Autodesk Inventor part; units mm, degrees
(part 2 of 6)
  line L456 (38.3615, -15.9793) -> (38.1514, -15.9793) construction
  line L457 (38.1514, -15.9793) -> (38.3134, -15.1333) construction
  line L458 (38.3134, -15.1333) -> (38.3374, -15.0013) construction
  spline S134 degree 3 poles (38.3374, -15.0013) (38.3735, -14.7674) (38.3914, -14.4554) (38.5415, -14.2694) knots 58 58 58 58 59 59 59 59
  line L459 (38.3374, -15.0013) -> (38.3735, -14.7674) construction
  line L460 (38.3735, -14.7674) -> (38.3914, -14.4554) construction
  line L461 (38.3914, -14.4554) -> (38.5415, -14.2694) construction
  spline S135 degree 3 poles (38.5415, -14.2694) (38.5774, -14.2214) (38.985, -13.6999) (38.9854, -13.6994) knots 59 59 59 59 60 60 60 60
  line L462 (38.5415, -14.2694) -> (38.5774, -14.2214) construction
  line L463 (38.5774, -14.2214) -> (38.9854, -13.6994) construction
  line L464 (38.9854, -13.6994) -> (38.9854, -13.6994) construction
  spline S136 degree 3 poles (38.9854, -13.6994) (38.9734, -13.6934) (38.9255, -13.7534) (38.8954, -13.7894) knots 60 60 60 60 61 61 61 61
  line L465 (38.9854, -13.6994) -> (38.9734, -13.6934) construction
  line L466 (38.9734, -13.6934) -> (38.9255, -13.7534) construction
  line L467 (38.9255, -13.7534) -> (38.8954, -13.7894) construction
  spline S137 degree 3 poles (38.8954, -13.7894) (38.8954, -13.7954) (38.8895, -13.8014) (38.8894, -13.8014) knots 61 61 61 61 62 62 62 62
  line L468 (38.8954, -13.7894) -> (38.8954, -13.7954) construction
  line L469 (38.8954, -13.7954) -> (38.8894, -13.8014) construction
  line L470 (38.8894, -13.8014) -> (38.8894, -13.8014) construction
  spline S138 degree 3 poles (38.8894, -13.8014) (38.8835, -13.8134) (38.8774, -13.8194) (38.8774, -13.8194) knots 62 62 62 62 63 63 63 63
  line L471 (38.8894, -13.8014) -> (38.8835, -13.8134) construction
  line L472 (38.8835, -13.8134) -> (38.8774, -13.8194) construction
  line L473 (38.8774, -13.8194) -> (38.8774, -13.8194) construction
  spline S139 degree 3 poles (38.8774, -13.8194) (38.8774, -13.8134) (38.8835, -13.8074) (38.8894, -13.8014) knots 63 63 63 63 64 64 64 64
  line L474 (38.8774, -13.8194) -> (38.8774, -13.8134) construction
  line L475 (38.8774, -13.8134) -> (38.8835, -13.8074) construction
  line L476 (38.8835, -13.8074) -> (38.8894, -13.8014) construction
  line L477 (38.8894, -13.8014) -> (38.8954, -13.7894)
  line L478 (38.8954, -13.7894) -> (39.1534, -13.4414)
  line L479 (39.1534, -13.4414) -> (39.1714, -13.4174)
  line L480 (39.1714, -13.4174) -> (39.2194, -13.3514)
  spline S140 degree 3 poles (39.2194, -13.3514) (39.2254, -13.3574) (39.2194, -13.3694) (39.2134, -13.3814) knots 68 68 68 68 69 69 69 69
  line L481 (39.2194, -13.3514) -> (39.2254, -13.3574) construction
  line L482 (39.2254, -13.3574) -> (39.2194, -13.3694) construction
  line L483 (39.2194, -13.3694) -> (39.2134, -13.3814) construction
  line L484 (39.2134, -13.3814) -> (39.2675, -13.3214)
  line L485 (39.2675, -13.3214) -> (39.4234, -13.1174)
  spline S141 degree 3 poles (39.4234, -13.1174) (39.5374, -12.9554) (39.6454, -12.7814) (39.7474, -12.6134) knots 71 71 71 71 72 72 72 72
  line L486 (39.4234, -13.1174) -> (39.5374, -12.9554) construction
  line L487 (39.5374, -12.9554) -> (39.6454, -12.7814) construction
  line L488 (39.6454, -12.7814) -> (39.7474, -12.6134) construction
  spline S142 degree 3 poles (39.7474, -12.6134) (39.9094, -12.3374) (40.1314, -11.9414) (40.0114, -11.6054) knots 72 72 72 72 73 73 73 73
  line L489 (39.7474, -12.6134) -> (39.9094, -12.3374) construction
  line L490 (39.9094, -12.3374) -> (40.1314, -11.9414) construction
  line L491 (40.1314, -11.9414) -> (40.0114, -11.6054) construction
  spline S143 degree 3 poles (40.0114, -11.6054) (39.9214, -11.3594) (39.5914, -11.3114) (39.3694, -11.3954) knots 73 73 73 73 74 74 74 74
  line L492 (40.0114, -11.6054) -> (39.9214, -11.3594) construction
  line L493 (39.9214, -11.3594) -> (39.5914, -11.3114) construction
  line L494 (39.5914, -11.3114) -> (39.3694, -11.3954) construction
  spline S144 degree 3 poles (39.3694, -11.3954) (39.2074, -11.4554) (39.0695, -11.5814) (38.9554, -11.7134) knots 74 74 74 74 75 75 75 75
  line L495 (39.3694, -11.3954) -> (39.2074, -11.4554) construction
  line L496 (39.2074, -11.4554) -> (39.0695, -11.5814) construction
  line L497 (39.0695, -11.5814) -> (38.9554, -11.7134) construction
  spline S145 degree 3 poles (38.9554, -11.7134) (38.8954, -11.7914) (38.8354, -11.8769) (38.7815, -11.9669) knots 75 75 75 75 76 76 76 76
  line L498 (38.9554, -11.7134) -> (38.8954, -11.7914) construction
  line L499 (38.8954, -11.7914) -> (38.8354, -11.8769) construction
  line L500 (38.8354, -11.8769) -> (38.7815, -11.9669) construction
  spline S146 degree 3 poles (38.7815, -11.9669) (38.7634, -11.9909) (38.6855, -12.1667) (38.6674, -12.2083) knots 76 76 76 76 77 77 77 77
  line L501 (38.7815, -11.9669) -> (38.7634, -11.9909) construction
  line L502 (38.7634, -11.9909) -> (38.6855, -12.1667) construction
  line L503 (38.6855, -12.1667) -> (38.6674, -12.2083) construction
  line L504 (38.6674, -12.2083) -> (38.6735, -12.2083)
  spline S147 degree 3 poles (38.6735, -12.2083) (38.6375, -12.2917) (38.6014, -12.3389) (38.5774, -12.4049) knots 78 78 78 78 79 79 79 79
  line L505 (38.6735, -12.2083) -> (38.6375, -12.2917) construction
  line L506 (38.6375, -12.2917) -> (38.6014, -12.3389) construction
  line L507 (38.6014, -12.3389) -> (38.5774, -12.4049) construction
  spline S148 degree 3 poles (38.5774, -12.4049) (38.5894, -12.3569) (38.6195, -12.2601) (38.6434, -12.2421) knots 79 79 79 79 80 80 80 80
  line L508 (38.5774, -12.4049) -> (38.5894, -12.3569) construction
  line L509 (38.5894, -12.3569) -> (38.6195, -12.2601) construction
  line L510 (38.6195, -12.2601) -> (38.6434, -12.2421) construction
  spline S149 degree 3 poles (38.6434, -12.2421) (38.5955, -12.2781) (38.5535, -12.4518) (38.5415, -12.4698) knots 80 80 80 80 81 81 81 81
  line L511 (38.6434, -12.2421) -> (38.5955, -12.2781) construction
  line L512 (38.5955, -12.2781) -> (38.5535, -12.4518) construction
  line L513 (38.5535, -12.4518) -> (38.5415, -12.4698) construction
  spline S150 degree 3 poles (38.5415, -12.4698) (38.3134, -12.9678) (38.1155, -13.4716) (37.9715, -13.9996) knots 81 81 81 81 82 82 82 82
  line L514 (38.5415, -12.4698) -> (38.3134, -12.9678) construction
  line L515 (38.3134, -12.9678) -> (38.1155, -13.4716) construction
  line L516 (38.1155, -13.4716) -> (37.9715, -13.9996) construction
  spline S151 degree 3 poles (37.9715, -13.9996) (37.8094, -13.8136) (37.5515, -13.4955) (37.2695, -13.6095) knots 82 82 82 82 83 83 83 83
  line L517 (37.9715, -13.9996) -> (37.8094, -13.8136) construction
  line L518 (37.8094, -13.8136) -> (37.5515, -13.4955) construction
  line L519 (37.5515, -13.4955) -> (37.2695, -13.6095) construction
  spline S152 degree 3 poles (37.2695, -13.6095) (37.0355, -13.7054) (36.8615, -13.9514) (36.7415, -14.1674) knots 83 83 83 83 84 84 84 84
  line L520 (37.2695, -13.6095) -> (37.0355, -13.7054) construction
  line L521 (37.0355, -13.7054) -> (36.8615, -13.9514) construction
  line L522 (36.8615, -13.9514) -> (36.7415, -14.1674) construction
  spline S153 degree 3 poles (36.7415, -14.1674) (36.7197, -14.2061) (36.7017, -14.2451) (36.6852, -14.2842) knots 84 84 84 84 85 85 85 85
  line L523 (36.7415, -14.1674) -> (36.7197, -14.2061) construction
  line L524 (36.7197, -14.2061) -> (36.7017, -14.2451) construction
  line L525 (36.7017, -14.2451) -> (36.6852, -14.2842) construction
  spline S154 degree 3 poles (36.6852, -14.2842) (36.6202, -14.3421) (36.5497, -14.3987) (36.4895, -14.4554) knots 85 85 85 85 86 86 86 86
  line L526 (36.6852, -14.2842) -> (36.6202, -14.3421) construction
  line L527 (36.6202, -14.3421) -> (36.5497, -14.3987) construction
  line L528 (36.5497, -14.3987) -> (36.4895, -14.4554) construction
  spline S155 degree 3 poles (36.4895, -14.4554) (36.3515, -14.5754) (36.2135, -14.7014) (36.0695, -14.8153) knots 86 86 86 86 87 87 87 87
  line L529 (36.4895, -14.4554) -> (36.3515, -14.5754) construction
  line L530 (36.3515, -14.5754) -> (36.2135, -14.7014) construction
  line L531 (36.2135, -14.7014) -> (36.0695, -14.8153) construction
  spline S156 degree 3 poles (36.0695, -14.8153) (35.9975, -14.8753) (35.9075, -14.9594) (35.8175, -14.9893) knots 87 87 87 87 88 88 88 88
  line L532 (36.0695, -14.8153) -> (35.9975, -14.8753) construction
  line L533 (35.9975, -14.8753) -> (35.9075, -14.9594) construction
  line L534 (35.9075, -14.9594) -> (35.8175, -14.9893) construction
  spline S157 degree 3 poles (35.8175, -14.9893) (35.8055, -14.9953) (35.7635, -15.0013) (35.7635, -15.0073) knots 88 88 88 88 89 89 89 89
  line L535 (35.8175, -14.9893) -> (35.8055, -14.9953) construction
  line L536 (35.8055, -14.9953) -> (35.7635, -15.0013) construction
  line L537 (35.7635, -15.0013) -> (35.7635, -15.0073) construction
  line L538 (35.7635, -15.0073) -> (35.7575, -15.0013)
  spline S158 degree 3 poles (35.7575, -15.0013) (35.7575, -15.0012) (35.7515, -14.9054) (35.7575, -14.8994) knots 90 90 90 90 91 91 91 91
  line L539 (35.7575, -15.0013) -> (35.7575, -15.0013) construction
  line L540 (35.7575, -15.0013) -> (35.7515, -14.9054) construction
  line L541 (35.7515, -14.9054) -> (35.7575, -14.8994) construction
  spline S159 degree 3 poles (35.7575, -14.8994) (35.7635, -14.8214) (35.7875, -14.7433) (35.8115, -14.6713) knots 91 91 91 91 92 92 92 92
  line L542 (35.7575, -14.8994) -> (35.7635, -14.8214) construction
  line L543 (35.7635, -14.8214) -> (35.7875, -14.7433) construction
  line L544 (35.7875, -14.7433) -> (35.8115, -14.6713) construction
  spline S160 degree 3 poles (35.8115, -14.6713) (35.8175, -14.6593) (35.8835, -14.4554) (35.8715, -14.4554) knots 92 92 92 92 93 93 93 93
  line L545 (35.8115, -14.6713) -> (35.8175, -14.6593) construction
  line L546 (35.8175, -14.6593) -> (35.8835, -14.4554) construction
  line L547 (35.8835, -14.4554) -> (35.8715, -14.4554) construction
  line L548 (35.8715, -14.4554) -> (35.8415, -14.4914)
  spline S161 degree 3 poles (35.8415, -14.4914) (35.8775, -14.4194) (35.9255, -14.3474) (35.9675, -14.2694) knots 94 94 94 94 95 95 95 95
  line L549 (35.8415, -14.4914) -> (35.8775, -14.4194) construction
  line L550 (35.8775, -14.4194) -> (35.9255, -14.3474) construction
  line L551 (35.9255, -14.3474) -> (35.9675, -14.2694) construction
  spline S162 degree 3 poles (35.9675, -14.2694) (35.8715, -14.3594) (35.8055, -14.4614) (35.7575, -14.5874) knots 95 95 95 95 96 96 96 96
  line L552 (35.9675, -14.2694) -> (35.8715, -14.3594) construction
  line L553 (35.8715, -14.3594) -> (35.8055, -14.4614) construction
  line L554 (35.8055, -14.4614) -> (35.7575, -14.5874) construction
  spline S163 degree 3 poles (35.7575, -14.5874) (35.7335, -14.6474) (35.6675, -14.7554) (35.6555, -14.8454) knots 96 96 96 96 97 97 97 97
  line L555 (35.7575, -14.5874) -> (35.7335, -14.6474) construction
  line L556 (35.7335, -14.6474) -> (35.6675, -14.7554) construction
  line L557 (35.6675, -14.7554) -> (35.6555, -14.8454) construction
  spline S164 degree 3 poles (35.6555, -14.8454) (35.6675, -14.7134) (35.7575, -14.5393) (35.7995, -14.4614) knots 97 97 97 97 98 98 98 98
  line L558 (35.6555, -14.8454) -> (35.6675, -14.7134) construction
  line L559 (35.6675, -14.7134) -> (35.7575, -14.5393) construction
  line L560 (35.7575, -14.5393) -> (35.7995, -14.4614) construction
  spline S165 degree 3 poles (35.7995, -14.4614) (35.8595, -14.3354) (35.9255, -14.1914) (36.0035, -14.0714) knots 98 98 98 98 99 99 99 99
  line L561 (35.7995, -14.4614) -> (35.8595, -14.3354) construction
  line L562 (35.8595, -14.3354) -> (35.9255, -14.1914) construction
  line L563 (35.9255, -14.1914) -> (36.0035, -14.0714) construction
  spline S166 degree 3 poles (36.0035, -14.0714) (36.1475, -13.8554) (36.4595, -13.6574) (36.3635, -13.3574) knots 99 99 99 99 100 100 100 100
  line L564 (36.0035, -14.0714) -> (36.1475, -13.8554) construction
  line L565 (36.1475, -13.8554) -> (36.4595, -13.6574) construction
  line L566 (36.4595, -13.6574) -> (36.3635, -13.3574) construction
  spline S167 degree 3 poles (36.3635, -13.3574) (36.2795, -13.0754) (36.0575, -13.0694) (35.8835, -13.2314) knots 100 100 100 100 101 101 101 101
  line L567 (36.3635, -13.3574) -> (36.2795, -13.0754) construction
  line L568 (36.2795, -13.0754) -> (36.0575, -13.0694) construction
  line L569 (36.0575, -13.0694) -> (35.8835, -13.2314) construction
  spline S168 degree 3 poles (35.8835, -13.2314) (35.7995, -13.3094) (35.0855, -14.2214) (35.1036, -14.2334) knots 101 101 101 101 102 102 102 102
  line L570 (35.8835, -13.2314) -> (35.7995, -13.3094) construction
  line L571 (35.7995, -13.3094) -> (35.0855, -14.2214) construction
  line L572 (35.0855, -14.2214) -> (35.1036, -14.2334) construction
  spline S169 degree 3 poles (35.1036, -14.2334) (35.1036, -14.2333) (35.1635, -14.1614) (35.2415, -14.0594) knots 102 102 102 102 103 103 103 103
  line L573 (35.1036, -14.2334) -> (35.1036, -14.2334) construction
  line L574 (35.1036, -14.2334) -> (35.1635, -14.1614) construction
  line L575 (35.1635, -14.1614) -> (35.2415, -14.0594) construction
  line L576 (35.2415, -14.0594) -> (34.8875, -14.5754)
  spline S170 degree 3 poles (34.8875, -14.5754) (34.8816, -14.5754) (34.9476, -14.4733) (34.9415, -14.4673) knots 104 104 104 104 105 105 105 105
  line L577 (34.8875, -14.5754) -> (34.8816, -14.5754) construction
  line L578 (34.8816, -14.5754) -> (34.9476, -14.4733) construction
  line L579 (34.9476, -14.4733) -> (34.9415, -14.4673) construction
  spline S171 degree 3 poles (34.9415, -14.4673) (34.9355, -14.4614) (34.8936, -14.5034) (34.8875, -14.5273) knots 105 105 105 105 106 106 106 106
  line L580 (34.9415, -14.4673) -> (34.9355, -14.4614) construction
  line L581 (34.9355, -14.4614) -> (34.8936, -14.5034) construction
  line L582 (34.8936, -14.5034) -> (34.8875, -14.5273) construction
  spline S172 degree 3 poles (34.8875, -14.5273) (34.8995, -14.4013) (34.9415, -14.2753) (34.9535, -14.1494) knots 106 106 106 106 107 107 107 107
  line L583 (34.8875, -14.5273) -> (34.8995, -14.4013) construction
  line L584 (34.8995, -14.4013) -> (34.9415, -14.2753) construction
  line L585 (34.9415, -14.2753) -> (34.9535, -14.1494) construction
  spline S173 degree 3 poles (34.9535, -14.1494) (34.9596, -14.1014) (34.9535, -14.0654) (34.9655, -14.0174) knots 107 107 107 107 108 108 108 108
  line L586 (34.9535, -14.1494) -> (34.9596, -14.1014) construction
  line L587 (34.9596, -14.1014) -> (34.9535, -14.0654) construction
  line L588 (34.9535, -14.0654) -> (34.9655, -14.0174) construction
  spline S174 degree 3 poles (34.9655, -14.0174) (34.9895, -13.9394) (35.0135, -13.8554) (35.0496, -13.7894) knots 108 108 108 108 109 109 109 109
  line L589 (34.9655, -14.0174) -> (34.9895, -13.9394) construction
  line L590 (34.9895, -13.9394) -> (35.0135, -13.8554) construction
  line L591 (35.0135, -13.8554) -> (35.0496, -13.7894) construction
  spline S175 degree 3 poles (35.0496, -13.7894) (35.0735, -13.7414) (35.1215, -13.6994) (35.1335, -13.6514) knots 109 109 109 109 110 110 110 110
  line L592 (35.0496, -13.7894) -> (35.0735, -13.7414) construction
  line L593 (35.0735, -13.7414) -> (35.1215, -13.6994) construction
  line L594 (35.1215, -13.6994) -> (35.1335, -13.6514) construction
  spline S176 degree 3 poles (35.1335, -13.6514) (35.1576, -13.5734) (35.1515, -13.5434) (35.2055, -13.4774) knots 110 110 110 110 111 111 111 111
  line L595 (35.1335, -13.6514) -> (35.1576, -13.5734) construction
  line L596 (35.1576, -13.5734) -> (35.1515, -13.5434) construction
  line L597 (35.1515, -13.5434) -> (35.2055, -13.4774) construction
  spline S177 degree 3 poles (35.2055, -13.4774) (35.2535, -13.4174) (35.3255, -13.3574) (35.3676, -13.3034) knots 111 111 111 111 112 112 112 112
  line L598 (35.2055, -13.4774) -> (35.2535, -13.4174) construction
  line L599 (35.2535, -13.4174) -> (35.3255, -13.3574) construction
  line L600 (35.3255, -13.3574) -> (35.3676, -13.3034) construction
  spline S178 degree 3 poles (35.3676, -13.3034) (35.4695, -13.1534) (35.2955, -13.0514) (35.1995, -13.0334) knots 112 112 112 112 113 113 113 113
  line L601 (35.3676, -13.3034) -> (35.4695, -13.1534) construction
  line L602 (35.4695, -13.1534) -> (35.2955, -13.0514) construction
  line L603 (35.2955, -13.0514) -> (35.1995, -13.0334) construction
  spline S179 degree 3 poles (35.1995, -13.0334) (35.1215, -13.0214) (35.0435, -13.0154) (34.9716, -13.0574) knots 113 113 113 113 114 114 114 114
  line L604 (35.1995, -13.0334) -> (35.1215, -13.0214) construction
  line L605 (35.1215, -13.0214) -> (35.0435, -13.0154) construction
  line L606 (35.0435, -13.0154) -> (34.9716, -13.0574) construction
  spline S180 degree 3 poles (34.9716, -13.0574) (34.8936, -13.1054) (34.9115, -13.1474) (34.8936, -13.2134) knots 114 114 114 114 115 115 115 115
  line L607 (34.9716, -13.0574) -> (34.8936, -13.1054) construction
  line L608 (34.8936, -13.1054) -> (34.9115, -13.1474) construction
  line L609 (34.9115, -13.1474) -> (34.8936, -13.2134) construction
  spline S181 degree 3 poles (34.8936, -13.2134) (34.8755, -13.2974) (34.8156, -13.3934) (34.7856, -13.4714) knots 115 115 115 115 116 116 116 116
  line L610 (34.8936, -13.2134) -> (34.8755, -13.2974) construction
  line L611 (34.8755, -13.2974) -> (34.8156, -13.3934) construction
  line L612 (34.8156, -13.3934) -> (34.7856, -13.4714) construction
  spline S182 degree 3 poles (34.7856, -13.4714) (34.7375, -13.5974) (34.6956, -13.7234) (34.6536, -13.8494) knots 116 116 116 116 117 117 117 117
  line L613 (34.7856, -13.4714) -> (34.7375, -13.5974) construction
  line L614 (34.7375, -13.5974) -> (34.6956, -13.7234) construction
  line L615 (34.6956, -13.7234) -> (34.6536, -13.8494) construction
  spline S183 degree 3 poles (34.6536, -13.8494) (34.6056, -13.9754) (34.5575, -14.0954) (34.5216, -14.2214) knots 117 117 117 117 118 118 118 118
  line L616 (34.6536, -13.8494) -> (34.6056, -13.9754) construction
  line L617 (34.6056, -13.9754) -> (34.5575, -14.0954) construction
  line L618 (34.5575, -14.0954) -> (34.5216, -14.2214) construction
  spline S184 degree 3 poles (34.5216, -14.2214) (34.4915, -14.3234) (34.4976, -14.4194) (34.4856, -14.5154) knots 118 118 118 118 119 119 119 119
  line L619 (34.5216, -14.2214) -> (34.4915, -14.3234) construction
  line L620 (34.4915, -14.3234) -> (34.4976, -14.4194) construction
  line L621 (34.4976, -14.4194) -> (34.4856, -14.5154) construction
  spline S185 degree 3 poles (34.4856, -14.5154) (34.4815, -14.5514) (34.4771, -14.5833) (34.4746, -14.6136) knots 119 119 119 119 120 120 120 120
  line L622 (34.4856, -14.5154) -> (34.4815, -14.5514) construction
  line L623 (34.4815, -14.5514) -> (34.4771, -14.5833) construction
  line L624 (34.4771, -14.5833) -> (34.4746, -14.6136) construction
  spline S186 degree 3 poles (34.4746, -14.6136) (34.3338, -14.8266) (34.1908, -15.0385) (34.0296, -15.2413) knots 120 120 120 120 121 121 121 121
  line L625 (34.4746, -14.6136) -> (34.3338, -14.8266) construction
  line L626 (34.3338, -14.8266) -> (34.1908, -15.0385) construction
  line L627 (34.1908, -15.0385) -> (34.0296, -15.2413) construction
  spline S187 degree 3 poles (34.0296, -15.2413) (33.4116, -16.0033) (33.8436, -14.6474) (33.7956, -14.6593) knots 121 121 121 121 122 122 122 122
  line L628 (34.0296, -15.2413) -> (33.4116, -16.0033) construction
  line L629 (33.4116, -16.0033) -> (33.8436, -14.6474) construction
  line L630 (33.8436, -14.6474) -> (33.7956, -14.6593) construction
  spline S188 degree 3 poles (33.7956, -14.6593) (33.7716, -14.6653) (33.7536, -14.7554) (33.7476, -14.7734) knots 122 122 122 122 123 123 123 123
  line L631 (33.7956, -14.6593) -> (33.7716, -14.6653) construction
  line L632 (33.7716, -14.6653) -> (33.7536, -14.7554) construction
  line L633 (33.7536, -14.7554) -> (33.7476, -14.7734) construction
  spline S189 degree 3 poles (33.7476, -14.7734) (33.7956, -14.5574) (33.8856, -14.2994) (33.9996, -14.0894) knots 123 123 123 123 124 124 124 124
  line L634 (33.7476, -14.7734) -> (33.7956, -14.5574) construction
  line L635 (33.7956, -14.5574) -> (33.8856, -14.2994) construction
  line L636 (33.8856, -14.2994) -> (33.9996, -14.0894) construction
  spline S190 degree 3 poles (33.9996, -14.0894) (34.0656, -13.9574) (34.1436, -13.8494) (34.0236, -13.7054) knots 124 124 124 124 125 125 125 125
  line L637 (33.9996, -14.0894) -> (34.0656, -13.9574) construction
  line L638 (34.0656, -13.9574) -> (34.1436, -13.8494) construction
  line L639 (34.1436, -13.8494) -> (34.0236, -13.7054) construction
  spline S191 degree 3 poles (34.0236, -13.7054) (33.8016, -13.4354) (33.5436, -13.6814) (33.3996, -13.8674) knots 125 125 125 125 126 126 126 126
  line L640 (34.0236, -13.7054) -> (33.8016, -13.4354) construction
  line L641 (33.8016, -13.4354) -> (33.5436, -13.6814) construction
  line L642 (33.5436, -13.6814) -> (33.3996, -13.8674) construction
  spline S192 degree 3 poles (33.3996, -13.8674) (33.3396, -13.6394) (33.2196, -13.3034) (32.9256, -13.3034) (32.7936, -13.3034) (32.7156, -13.3694) (32.6256, -13.4474) knots 126 126 126 126 127 127 127 128 128 128 128
  line L643 (33.3996, -13.8674) -> (33.3396, -13.6394) construction
  line L644 (33.3396, -13.6394) -> (33.2196, -13.3034) construction
  line L645 (33.2196, -13.3034) -> (32.9256, -13.3034) construction
  line L646 (32.9256, -13.3034) -> (32.7936, -13.3034) construction
  line L647 (32.7936, -13.3034) -> (32.7156, -13.3694) construction
  line L648 (32.7156, -13.3694) -> (32.6256, -13.4474) construction
  spline S193 degree 3 poles (32.6256, -13.4474) (32.5716, -13.4834) (32.5296, -13.4894) (32.4816, -13.5314) knots 128 128 128 128 129 129 129 129
  line L649 (32.6256, -13.4474) -> (32.5716, -13.4834) construction
  line L650 (32.5716, -13.4834) -> (32.5296, -13.4894) construction
  line L651 (32.5296, -13.4894) -> (32.4816, -13.5314) construction
  spline S194 degree 3 poles (32.4816, -13.5314) (32.4036, -13.5854) (32.3496, -13.6694) (32.2956, -13.7414) knots 129 129 129 129 130 130 130 130
  line L652 (32.4816, -13.5314) -> (32.4036, -13.5854) construction
  line L653 (32.4036, -13.5854) -> (32.3496, -13.6694) construction
  line L654 (32.3496, -13.6694) -> (32.2956, -13.7414) construction
  spline S195 degree 3 poles (32.2956, -13.7414) (32.0916, -14.0414) (31.9476, -14.4194) (31.8816, -14.7674) knots 130 130 130 130 131 131 131 131
  line L655 (32.2956, -13.7414) -> (32.0916, -14.0414) construction
  line L656 (32.0916, -14.0414) -> (31.9476, -14.4194) construction
  line L657 (31.9476, -14.4194) -> (31.8816, -14.7674) construction
  spline S196 degree 3 poles (31.8816, -14.7674) (31.8516, -14.9353) (31.8396, -15.1213) (31.8876, -15.2893) knots 131 131 131 131 132 132 132 132
  line L658 (31.8816, -14.7674) -> (31.8516, -14.9353) construction
  line L659 (31.8516, -14.9353) -> (31.8396, -15.1213) construction
  line L660 (31.8396, -15.1213) -> (31.8876, -15.2893) construction
  spline S197 degree 3 poles (31.8876, -15.2893) (31.9176, -15.3853) (32.0256, -15.6013) (32.1636, -15.5833) knots 132 132 132 132 133 133 133 133
  line L661 (31.8876, -15.2893) -> (31.9176, -15.3853) construction
  line L662 (31.9176, -15.3853) -> (32.0256, -15.6013) construction
  line L663 (32.0256, -15.6013) -> (32.1636, -15.5833) construction
  spline S198 degree 3 poles (32.1636, -15.5833) (32.1696, -15.5833) (32.1576, -15.5773) (32.1396, -15.5653) knots 133 133 133 133 134 134 134 134
  line L664 (32.1636, -15.5833) -> (32.1696, -15.5833) construction
  line L665 (32.1696, -15.5833) -> (32.1576, -15.5773) construction
  line L666 (32.1576, -15.5773) -> (32.1396, -15.5653) construction
  spline S199 degree 3 poles (32.1396, -15.5653) (32.2236, -15.5893) (32.3196, -15.5773) (32.3916, -15.5293) knots 134 134 134 134 135 135 135 135
  line L667 (32.1396, -15.5653) -> (32.2236, -15.5893) construction
  line L668 (32.2236, -15.5893) -> (32.3196, -15.5773) construction
  line L669 (32.3196, -15.5773) -> (32.3916, -15.5293) construction
  spline S200 degree 3 poles (32.3916, -15.5293) (32.3976, -15.5413) (32.3257, -15.5713) (32.3256, -15.5713) knots 135 135 135 135 136 136 136 136
  line L670 (32.3916, -15.5293) -> (32.3976, -15.5413) construction
  line L671 (32.3976, -15.5413) -> (32.3256, -15.5713) construction
  line L672 (32.3256, -15.5713) -> (32.3256, -15.5713) construction
  spline S201 degree 3 poles (32.3256, -15.5713) (32.3916, -15.6733) (32.8836, -15.0793) (32.9196, -15.0253) knots 136 136 136 136 137 137 137 137
  line L673 (32.3256, -15.5713) -> (32.3916, -15.6733) construction
  line L674 (32.3916, -15.6733) -> (32.8836, -15.0793) construction
  line L675 (32.8836, -15.0793) -> (32.9196, -15.0253) construction
  spline S202 degree 3 poles (32.9196, -15.0253) (32.9976, -14.9173) (33.0516, -14.8033) (33.1236, -14.6894) knots 137 137 137 137 138 138 138 138
  line L676 (32.9196, -15.0253) -> (32.9976, -14.9173) construction
  line L677 (32.9976, -14.9173) -> (33.0516, -14.8033) construction
  line L678 (33.0516, -14.8033) -> (33.1236, -14.6894) construction
  spline S203 degree 3 poles (33.1236, -14.6894) (33.1776, -14.6053) (33.2616, -14.4974) (33.3216, -14.4073) knots 138 138 138 138 139 139 139 139
  line L679 (33.1236, -14.6894) -> (33.1776, -14.6053) construction
  line L680 (33.1776, -14.6053) -> (33.2616, -14.4974) construction
  line L681 (33.2616, -14.4974) -> (33.3216, -14.4073) construction
  spline S204 degree 3 poles (33.3216, -14.4073) (33.3156, -14.4494) (33.3156, -14.5033) (33.3156, -14.5034) knots 139 139 139 139 140 140 140 140
  line L682 (33.3216, -14.4073) -> (33.3156, -14.4494) construction
  line L683 (33.3156, -14.4494) -> (33.3156, -14.5034) construction
  line L684 (33.3156, -14.5034) -> (33.3156, -14.5034) construction
  spline S205 degree 3 poles (33.3156, -14.5034) (33.2076, -14.8454) (33.1056, -15.2173) (33.2496, -15.5713) knots 140 140 140 140 141 141 141 141
  line L685 (33.3156, -14.5034) -> (33.2076, -14.8454) construction
  line L686 (33.2076, -14.8454) -> (33.1056, -15.2173) construction
  line L687 (33.1056, -15.2173) -> (33.2496, -15.5713) construction
  spline S206 degree 3 poles (33.2496, -15.5713) (33.3156, -15.7513) (33.4776, -15.9193) (33.6816, -15.8833) knots 141 141 141 141 142 142 142 142
  line L688 (33.2496, -15.5713) -> (33.3156, -15.7513) construction
  line L689 (33.3156, -15.7513) -> (33.4776, -15.9193) construction
  line L690 (33.4776, -15.9193) -> (33.6816, -15.8833) construction
  spline S207 degree 3 poles (33.6816, -15.8833) (33.8616, -15.8533) (34.0116, -15.6793) (34.1196, -15.5413) knots 142 142 142 142 143 143 143 143
  line L691 (33.6816, -15.8833) -> (33.8616, -15.8533) construction
  line L692 (33.8616, -15.8533) -> (34.0116, -15.6793) construction
  line L693 (34.0116, -15.6793) -> (34.1196, -15.5413) construction
  spline S208 degree 3 poles (34.1196, -15.5413) (34.2516, -15.3853) (34.3656, -15.2113) (34.4796, -15.0314) knots 143 143 143 143 144 144 144 144
  line L694 (34.1196, -15.5413) -> (34.2516, -15.3853) construction
  line L695 (34.2516, -15.3853) -> (34.3656, -15.2113) construction
  line L696 (34.3656, -15.2113) -> (34.4796, -15.0314) construction
  spline S209 degree 3 poles (34.4796, -15.0314) (34.5108, -14.9786) (34.5411, -14.9256) (34.5709, -14.8722) knots 144 144 144 144 145 145 145 145
  line L697 (34.4796, -15.0314) -> (34.5108, -14.9786) construction
  line L698 (34.5108, -14.9786) -> (34.5411, -14.9256) construction
  line L699 (34.5411, -14.9256) -> (34.5709, -14.8722) construction
  spline S210 degree 3 poles (34.5709, -14.8722) (34.6468, -14.9531) (34.7584, -15.0165) (34.8396, -14.9173) knots 145 145 145 145 146 146 146 146
  line L700 (34.5709, -14.8722) -> (34.6468, -14.9531) construction
  line L701 (34.6468, -14.9531) -> (34.7584, -15.0165) construction
  line L702 (34.7584, -15.0165) -> (34.8396, -14.9173) construction
  line L703 (34.8396, -14.9173) -> (34.8635, -14.9654)
  spline S211 degree 3 poles (34.8635, -14.9654) (34.9655, -14.7433) (35.1215, -14.5453) (35.2475, -14.3294) knots 147 147 147 147 148 148 148 148
  line L704 (34.8635, -14.9654) -> (34.9655, -14.7433) construction
  line L705 (34.9655, -14.7433) -> (35.1215, -14.5453) construction
  line L706 (35.1215, -14.5453) -> (35.2475, -14.3294) construction
  spline S212 degree 3 poles (35.2475, -14.3294) (35.3016, -14.2334) (35.3975, -14.1674) (35.4755, -14.0654) knots 148 148 148 148 149 149 149 149
  line L707 (35.2475, -14.3294) -> (35.3016, -14.2334) construction
  line L708 (35.3016, -14.2334) -> (35.3975, -14.1674) construction
  line L709 (35.3975, -14.1674) -> (35.4755, -14.0654) construction
  spline S213 degree 3 poles (35.4755, -14.0654) (35.5835, -13.9214) (35.6795, -13.7774) (35.7995, -13.6394) knots 149 149 149 149 150 150 150 150
  line L710 (35.4755, -14.0654) -> (35.5835, -13.9214) construction
  line L711 (35.5835, -13.9214) -> (35.6795, -13.7774) construction
  line L712 (35.6795, -13.7774) -> (35.7995, -13.6394) construction
  spline S214 degree 3 poles (35.7995, -13.6394) (35.7815, -13.6694) (35.7035, -13.8074) (35.7095, -13.8134) knots 150 150 150 150 151 151 151 151
  line L713 (35.7995, -13.6394) -> (35.7815, -13.6694) construction
  line L714 (35.7815, -13.6694) -> (35.7035, -13.8074) construction
  line L715 (35.7035, -13.8074) -> (35.7095, -13.8134) construction
  spline S215 degree 3 poles (35.7095, -13.8134) (35.7215, -13.8074) (35.7275, -13.7954) (35.7395, -13.7834) knots 151 151 151 151 152 152 152 152
  line L716 (35.7095, -13.8134) -> (35.7215, -13.8074) construction
  line L717 (35.7215, -13.8074) -> (35.7275, -13.7954) construction
  line L718 (35.7275, -13.7954) -> (35.7395, -13.7834) construction
  line L719 (35.7395, -13.7834) -> (35.6555, -13.9514)
  spline S216 degree 3 poles (35.6555, -13.9514) (35.6495, -13.9454) (35.6795, -13.9034) (35.6675, -13.9034) knots 153 153 153 153 154 154 154 154
  line L720 (35.6555, -13.9514) -> (35.6495, -13.9454) construction
  line L721 (35.6495, -13.9454) -> (35.6795, -13.9034) construction
  line L722 (35.6795, -13.9034) -> (35.6675, -13.9034) construction
  spline S217 degree 3 poles (35.6675, -13.9034) (35.6255, -13.8914) (35.4995, -14.2274) (35.4875, -14.2574) knots 154 154 154 154 155 155 155 155
  line L723 (35.6675, -13.9034) -> (35.6255, -13.8914) construction
  line L724 (35.6255, -13.8914) -> (35.4995, -14.2274) construction
  line L725 (35.4995, -14.2274) -> (35.4875, -14.2574) construction
  spline S218 degree 3 poles (35.4875, -14.2574) (35.4455, -14.3894) (35.4395, -14.5094) (35.4275, -14.6474) knots 155 155 155 155 156 156 156 156
  line L726 (35.4875, -14.2574) -> (35.4455, -14.3894) construction
  line L727 (35.4455, -14.3894) -> (35.4395, -14.5094) construction
  line L728 (35.4395, -14.5094) -> (35.4275, -14.6474) construction
  spline S219 degree 3 poles (35.4275, -14.6474) (35.4215, -14.7134) (35.4095, -14.7794) (35.4095, -14.8454) (35.4095, -14.9113) (35.4155, -14.9773) (35.4455, -15.0433) knots 156 156 156 156 157 157 157 158 158 158 158
  line L729 (35.4275, -14.6474) -> (35.4215, -14.7134) construction
  line L730 (35.4215, -14.7134) -> (35.4095, -14.7794) construction
  line L731 (35.4095, -14.7794) -> (35.4095, -14.8454) construction
  line L732 (35.4095, -14.8454) -> (35.4095, -14.9113) construction
  line L733 (35.4095, -14.9113) -> (35.4155, -14.9773) construction
  line L734 (35.4155, -14.9773) -> (35.4455, -15.0433) construction
  spline S220 degree 3 poles (35.4455, -15.0433) (35.4635, -15.0793) (35.4875, -15.1273) (35.5175, -15.1573) knots 158 158 158 158 159 159 159 159
  line L735 (35.4455, -15.0433) -> (35.4635, -15.0793) construction
  line L736 (35.4635, -15.0793) -> (35.4875, -15.1273) construction
  line L737 (35.4875, -15.1273) -> (35.5175, -15.1573) construction
  spline S221 degree 3 poles (35.5175, -15.1573) (35.5235, -15.1573) (35.5895, -15.2173) (35.5595, -15.1693) knots 159 159 159 159 160 160 160 160
  line L738 (35.5175, -15.1573) -> (35.5235, -15.1573) construction
  line L739 (35.5235, -15.1573) -> (35.5895, -15.2173) construction
  line L740 (35.5895, -15.2173) -> (35.5595, -15.1693) construction
  line L741 (35.5595, -15.1693) -> (35.5955, -15.2053)
  line L742 (35.5955, -15.2053) -> (35.5775, -15.1933)
  spline S222 degree 3 poles (35.5775, -15.1933) (35.5715, -15.2233) (35.7935, -15.3433) (35.8295, -15.3553) knots 162 162 162 162 163 163 163 163
  line L743 (35.5775, -15.1933) -> (35.5715, -15.2233) construction
  line L744 (35.5715, -15.2233) -> (35.7935, -15.3433) construction
  line L745 (35.7935, -15.3433) -> (35.8295, -15.3553) construction
  spline S223 degree 3 poles (35.8295, -15.3553) (35.9975, -15.4093) (36.1775, -15.2173) (36.2855, -15.1034) knots 163 163 163 163 164 164 164 164
  line L746 (35.8295, -15.3553) -> (35.9975, -15.4093) construction
  line L747 (35.9975, -15.4093) -> (36.1775, -15.2173) construction
  line L748 (36.1775, -15.2173) -> (36.2855, -15.1034) construction
  spline S224 degree 3 poles (36.2855, -15.1034) (36.3553, -15.0278) (36.4194, -14.9464) (36.482, -14.8636) knots 164 164 164 164 165 165 165 165
  line L749 (36.2855, -15.1034) -> (36.3553, -15.0278) construction
  line L750 (36.3553, -15.0278) -> (36.4194, -14.9464) construction
  line L751 (36.4194, -14.9464) -> (36.482, -14.8636) construction
  spline S225 degree 3 poles (36.482, -14.8636) (36.3795, -15.2029) (36.3747, -15.7262) (36.7895, -15.8113) knots 165 165 165 165 166 166 166 166
  line L752 (36.482, -14.8636) -> (36.3795, -15.2029) construction
  line L753 (36.3795, -15.2029) -> (36.3747, -15.7262) construction
  line L754 (36.3747, -15.7262) -> (36.7895, -15.8113) construction
  spline S226 degree 3 poles (36.7895, -15.8113) (36.9335, -15.8413) (37.0655, -15.7513) (37.1795, -15.6733) knots 166 166 166 166 167 167 167 167
  line L755 (36.7895, -15.8113) -> (36.9335, -15.8413) construction
  line L756 (36.9335, -15.8413) -> (37.0655, -15.7513) construction
  line L757 (37.0655, -15.7513) -> (37.1795, -15.6733) construction
  spline S227 degree 3 poles (37.1795, -15.6733) (37.3835, -15.5233) (37.5755, -15.3493) (37.7555, -15.1693) knots 167 167 167 167 168 168 168 168
  line L758 (37.1795, -15.6733) -> (37.3835, -15.5233) construction
  line L759 (37.3835, -15.5233) -> (37.5755, -15.3493) construction
  line L760 (37.5755, -15.3493) -> (37.7555, -15.1693) construction
  spline S228 degree 3 poles (37.7555, -15.1693) (37.7255, -15.4873) (37.6595, -15.9673) (37.9175, -16.2193) knots 168 168 168 168 169 169 169 169
  line L761 (37.7555, -15.1693) -> (37.7255, -15.4873) construction
  line L762 (37.7255, -15.4873) -> (37.6595, -15.9673) construction
  line L763 (37.6595, -15.9673) -> (37.9175, -16.2193) construction
  spline S229 degree 3 poles (37.9175, -16.2193) (38.2355, -16.5433) (38.5535, -16.1053) (38.7454, -15.8653) knots 169 169 169 169 170 170 170 170
  line L764 (37.9175, -16.2193) -> (38.2355, -16.5433) construction
  line L765 (38.2355, -16.5433) -> (38.5535, -16.1053) construction
  line L766 (38.5535, -16.1053) -> (38.7454, -15.8653) construction
  spline S230 degree 3 poles (38.7454, -15.8653) (38.9915, -15.5533) (39.1834, -15.2053) (39.4294, -14.9054) knots 170 170 170 170 171 171 171 171
  line L767 (38.7454, -15.8653) -> (38.9915, -15.5533) construction
  line L768 (38.9915, -15.5533) -> (39.1834, -15.2053) construction
  line L769 (39.1834, -15.2053) -> (39.4294, -14.9054) construction
  spline S231 degree 3 poles (39.4294, -14.9054) (39.5494, -14.7614) (39.6694, -14.6174) (39.7954, -14.4854) knots 171 171 171 171 172 172 172 172
  line L770 (39.4294, -14.9054) -> (39.5494, -14.7614) construction
  line L771 (39.5494, -14.7614) -> (39.6694, -14.6174) construction
  line L772 (39.6694, -14.6174) -> (39.7954, -14.4854) construction
  spline S232 degree 3 poles (39.7954, -14.4854) (39.807, -14.4738) (39.8199, -14.4619) (39.8337, -14.4497) knots 172 172 172 172 173 173 173 173
  line L773 (39.7954, -14.4854) -> (39.807, -14.4738) construction
  line L774 (39.807, -14.4738) -> (39.8199, -14.4619) construction
  line L775 (39.8199, -14.4619) -> (39.8337, -14.4497) construction
  spline S233 degree 3 poles (39.8337, -14.4497) (39.8284, -14.5014) (39.829, -14.5562) (39.8254, -14.5634) knots 173 173 173 173 174 174 174 174
  line L776 (39.8337, -14.4497) -> (39.8284, -14.5014) construction
  line L777 (39.8284, -14.5014) -> (39.829, -14.5562) construction
  line L778 (39.829, -14.5562) -> (39.8254, -14.5634) construction
  spline S234 degree 3 poles (39.8254, -14.5634) (39.7474, -14.8873) (39.6574, -15.2113) (39.6334, -15.5473) knots 174 174 174 174 175 175 175 175
  line L779 (39.8254, -14.5634) -> (39.7474, -14.8873) construction
  line L780 (39.7474, -14.8873) -> (39.6574, -15.2113) construction
  line L781 (39.6574, -15.2113) -> (39.6334, -15.5473) construction
  spline S235 degree 3 poles (39.6334, -15.5473) (39.6154, -15.8653) (39.6154, -16.2853) (39.8674, -16.5193) knots 175 175 175 175 176 176 176 176
  line L782 (39.6334, -15.5473) -> (39.6154, -15.8653) construction
  line L783 (39.6154, -15.8653) -> (39.6154, -16.2853) construction
  line L784 (39.6154, -16.2853) -> (39.8674, -16.5193) construction
  spline S236 degree 3 poles (39.8674, -16.5193) (40.1494, -16.7773) (40.4734, -16.6033) (40.7074, -16.3813) knots 176 176 176 176 177 177 177 177
  line L785 (39.8674, -16.5193) -> (40.1494, -16.7773) construction
  line L786 (40.1494, -16.7773) -> (40.4734, -16.6033) construction
  line L787 (40.4734, -16.6033) -> (40.7074, -16.3813) construction
  spline S237 degree 3 poles (40.7074, -16.3813) (40.9834, -16.1113) (41.2174, -15.7933) (41.4334, -15.4813) knots 177 177 177 177 178 178 178 178
  line L788 (40.7074, -16.3813) -> (40.9834, -16.1113) construction
  line L789 (40.9834, -16.1113) -> (41.2174, -15.7933) construction
  line L790 (41.2174, -15.7933) -> (41.4334, -15.4813) construction
  spline S238 degree 3 poles (41.4334, -15.4813) (41.5675, -15.2862) (41.6825, -15.0828) (41.7986, -14.8824) knots 178 178 178 178 179 179 179 179
  line L791 (41.4334, -15.4813) -> (41.5675, -15.2862) construction
  line L792 (41.5675, -15.2862) -> (41.6825, -15.0828) construction
  line L793 (41.6825, -15.0828) -> (41.7986, -14.8824) construction
  spline S239 degree 3 poles (41.7986, -14.8824) (41.791, -14.9297) (41.7834, -14.9773) (41.7754, -15.0253) knots 179 179 179 179 180 180 180 180
  line L794 (41.7986, -14.8824) -> (41.791, -14.9297) construction
  line L795 (41.791, -14.9297) -> (41.7834, -14.9773) construction
  line L796 (41.7834, -14.9773) -> (41.7754, -15.0253) construction
  spline S240 degree 3 poles (41.7754, -15.0253) (41.7454, -15.2053) (41.7274, -15.3733) (41.8234, -15.5413) knots 180 180 180 180 181 181 181 181
  line L797 (41.7754, -15.0253) -> (41.7454, -15.2053) construction
  line L798 (41.7454, -15.2053) -> (41.7274, -15.3733) construction
  line L799 (41.7274, -15.3733) -> (41.8234, -15.5413) construction
  spline S241 degree 3 poles (41.8234, -15.5413) (41.8174, -15.4813) (41.8054, -15.4273) (41.8054, -15.3733) (41.8054, -15.3433) (41.8174, -15.3133) (41.8174, -15.2893) (41.8174, -15.2773) (41.8054, -15.2413) (41.8054, -15.2233) (41.8054, -15.1693) (41.8174, -15.1273) (41.8294, -15.0733) knots 181 181 181 181 182 182 182 183 183 183 184 184 184 185 185 185 185
  line L800 (41.8234, -15.5413) -> (41.8174, -15.4813) construction
  line L801 (41.8174, -15.4813) -> (41.8054, -15.4273) construction
  line L802 (41.8054, -15.4273) -> (41.8054, -15.3733) construction
  line L803 (41.8054, -15.3733) -> (41.8054, -15.3433) construction
  line L804 (41.8054, -15.3433) -> (41.8174, -15.3133) construction
  line L805 (41.8174, -15.3133) -> (41.8174, -15.2893) construction
  line L806 (41.8174, -15.2893) -> (41.8174, -15.2773) construction
  line L807 (41.8174, -15.2773) -> (41.8054, -15.2413) construction
  line L808 (41.8054, -15.2413) -> (41.8054, -15.2233) construction
  line L809 (41.8054, -15.2233) -> (41.8054, -15.1693) construction
  line L810 (41.8054, -15.1693) -> (41.8174, -15.1273) construction
  line L811 (41.8174, -15.1273) -> (41.8294, -15.0733) construction
  spline S242 degree 3 poles (41.8294, -15.0733) (41.8354, -15.0193) (41.8294, -14.9654) (41.8354, -14.9113) knots 185 185 185 185 186 186 186 186
  line L812 (41.8294, -15.0733) -> (41.8354, -15.0193) construction
  line L813 (41.8354, -15.0193) -> (41.8294, -14.9654) construction
  line L814 (41.8294, -14.9654) -> (41.8354, -14.9113) construction
  spline S243 degree 3 poles (41.8354, -14.9113) (41.8414, -14.8513) (41.8654, -14.8033) (41.8894, -14.7493) knots 186 186 186 186 187 187 187 187
  line L815 (41.8354, -14.9113) -> (41.8414, -14.8513) construction
  line L816 (41.8414, -14.8513) -> (41.8654, -14.8033) construction
  line L817 (41.8654, -14.8033) -> (41.8894, -14.7493) construction
  spline S244 degree 3 poles (41.8894, -14.7493) (41.8954, -14.7333) (41.8999, -14.7179) (41.9042, -14.7027) knots 187 187 187 187 188 188 188 188
  line L818 (41.8894, -14.7493) -> (41.8954, -14.7333) construction
  line L819 (41.8954, -14.7333) -> (41.8999, -14.7179) construction
  line L820 (41.8999, -14.7179) -> (41.9042, -14.7027) construction
  spline S245 degree 3 poles (41.9042, -14.7027) (41.9216, -14.6737) (41.9393, -14.6449) (41.9571, -14.6162) knots 188 188 188 188 189 189 189 189
  line L821 (41.9042, -14.7027) -> (41.9216, -14.6737) construction
  line L822 (41.9216, -14.6737) -> (41.9393, -14.6449) construction
  line L823 (41.9393, -14.6449) -> (41.9571, -14.6162) construction
  spline S246 degree 3 poles (41.9571, -14.6162) (41.9565, -14.6591) (41.9588, -14.7022) (41.9554, -14.7433) knots 189 189 189 189 190 190 190 190
  line L824 (41.9571, -14.6162) -> (41.9565, -14.6591) construction
  line L825 (41.9565, -14.6591) -> (41.9588, -14.7022) construction
  line L826 (41.9588, -14.7022) -> (41.9554, -14.7433) construction
  spline S247 degree 3 poles (41.9554, -14.7433) (41.9434, -14.8214) (41.9194, -14.8994) (41.9074, -14.9833) knots 190 190 190 190 191 191 191 191
  line L827 (41.9554, -14.7433) -> (41.9434, -14.8214) construction
  line L828 (41.9434, -14.8214) -> (41.9194, -14.8994) construction
  line L829 (41.9194, -14.8994) -> (41.9074, -14.9833) construction
  spline S248 degree 3 poles (41.9074, -14.9833) (41.8954, -15.0613) (41.8594, -15.1333) (41.8474, -15.2113) knots 191 191 191 191 192 192 192 192
  line L830 (41.9074, -14.9833) -> (41.8954, -15.0613) construction
  line L831 (41.8954, -15.0613) -> (41.8594, -15.1333) construction
  line L832 (41.8594, -15.1333) -> (41.8474, -15.2113) construction
  spline S249 degree 3 poles (41.8474, -15.2113) (41.8354, -15.2833) (41.8114, -15.3373) (41.8174, -15.4093) knots 192 192 192 192 193 193 193 193
  line L833 (41.8474, -15.2113) -> (41.8354, -15.2833) construction
  line L834 (41.8354, -15.2833) -> (41.8114, -15.3373) construction
  line L835 (41.8114, -15.3373) -> (41.8174, -15.4093) construction
  spline S250 degree 3 poles (41.8174, -15.4093) (41.8174, -15.4513) (41.8234, -15.4933) (41.8294, -15.5293) knots 193 193 193 193 194 194 194 194
  line L836 (41.8174, -15.4093) -> (41.8174, -15.4513) construction
  line L837 (41.8174, -15.4513) -> (41.8234, -15.4933) construction
  line L838 (41.8234, -15.4933) -> (41.8294, -15.5293) construction
  spline S251 degree 3 poles (41.8294, -15.5293) (41.8354, -15.5773) (41.8654, -15.6073) (41.8954, -15.6433) knots 194 194 194 194 195 195 195 195
  line L839 (41.8294, -15.5293) -> (41.8354, -15.5773) construction
  line L840 (41.8354, -15.5773) -> (41.8654, -15.6073) construction
  line L841 (41.8654, -15.6073) -> (41.8954, -15.6433) construction
  spline S252 degree 3 poles (41.8954, -15.6433) (41.9974, -15.7633) (42.1354, -15.8593) (42.2914, -15.9013) knots 195 195 195 195 196 196 196 196
  line L842 (41.8954, -15.6433) -> (41.9974, -15.7633) construction
  line L843 (41.9974, -15.7633) -> (42.1354, -15.8593) construction
  line L844 (42.1354, -15.8593) -> (42.2914, -15.9013) construction
  spline S253 degree 3 poles (42.2914, -15.9013) (42.3994, -15.9313) (42.4954, -15.9253) (42.5974, -15.8713) knots 196 196 196 196 197 197 197 197
  line L845 (42.2914, -15.9013) -> (42.3994, -15.9313) construction
  line L846 (42.3994, -15.9313) -> (42.4954, -15.9253) construction
  line L847 (42.4954, -15.9253) -> (42.5974, -15.8713) construction
  spline S254 degree 3 poles (42.5974, -15.8713) (42.7414, -15.7933) (42.8674, -15.6733) (42.9753, -15.5593) knots 197 197 197 197 198 198 198 198
  line L848 (42.5974, -15.8713) -> (42.7414, -15.7933) construction
  line L849 (42.7414, -15.7933) -> (42.8674, -15.6733) construction
  line L850 (42.8674, -15.6733) -> (42.9753, -15.5593) construction
  spline S255 degree 3 poles (42.9753, -15.5593) (43.0774, -15.4453) (43.1554, -15.3193) (43.2454, -15.1993) knots 198 198 198 198 199 199 199 199
  line L851 (42.9753, -15.5593) -> (43.0774, -15.4453) construction
  line L852 (43.0774, -15.4453) -> (43.1554, -15.3193) construction
  line L853 (43.1554, -15.3193) -> (43.2454, -15.1993) construction
  spline S256 degree 3 poles (43.2454, -15.1993) (43.3293, -15.0913) (43.4314, -14.9893) (43.5153, -14.8813) knots 199 199 199 199 200 200 200 200
  line L854 (43.2454, -15.1993) -> (43.3293, -15.0913) construction
  line L855 (43.3293, -15.0913) -> (43.4314, -14.9893) construction
  line L856 (43.4314, -14.9893) -> (43.5153, -14.8813) construction
  line L857 (43.5153, -14.8813) -> (43.8394, -14.4614)
  line L858 (43.8394, -14.4614) -> (44.0253, -14.2063)
  spline S257 degree 3 poles (44.0253, -14.2063) (44.0553, -14.1703) (44.0725, -14.1667) (44.0485, -14.0833) knots 202 202 202 202 203 203 203 203
  line L859 (44.0253, -14.2063) -> (44.0553, -14.1703) construction
  line L860 (44.0553, -14.1703) -> (44.0725, -14.1667) construction
  line L861 (44.0725, -14.1667) -> (44.0485, -14.0833) construction
  spline S258 degree 3 poles (44.0485, -14.0833) (44.0485, -14.125) (44.0417, -14.125) (44.0417, -14.0833) knots 203 203 203 203 204 204 204 204
  line L862 (44.0485, -14.0833) -> (44.0485, -14.125) construction
  line L863 (44.0485, -14.125) -> (44.0417, -14.125) construction
  line L864 (44.0417, -14.125) -> (44.0417, -14.0833) construction
  spline S259 degree 3 poles (37.5215, -13.9394) (37.5035, -13.9574) (37.4855, -13.9814) (37.4735, -13.9814) (37.4795, -13.9814) (37.4975, -13.9574) (37.5215, -13.9394) knots 0 0 0 0 1 1 1 2 2 2 2
  line L865 (37.5215, -13.9394) -> (37.5035, -13.9574) construction
  line L866 (37.5035, -13.9574) -> (37.4855, -13.9814) construction
  line L867 (37.4855, -13.9814) -> (37.4735, -13.9814) construction
  line L868 (37.4735, -13.9814) -> (37.4795, -13.9814) construction
  line L869 (37.4795, -13.9814) -> (37.4975, -13.9574) construction
  line L870 (37.4975, -13.9574) -> (37.5215, -13.9394) construction
  spline S260 degree 3 poles (37.5215, -13.9394) (37.4975, -13.9574) (37.4795, -13.9814) (37.4735, -13.9814) (37.4855, -13.9814) (37.5035, -13.9574) (37.5215, -13.9394) knots 0 0 0 0 1 1 1 2 2 2 2
  line L871 (37.5215, -13.9394) -> (37.4975, -13.9574) construction
  line L872 (37.4975, -13.9574) -> (37.4795, -13.9814) construction
  line L873 (37.4795, -13.9814) -> (37.4735, -13.9814) construction
  line L874 (37.4735, -13.9814) -> (37.4855, -13.9814) construction
  line L875 (37.4855, -13.9814) -> (37.5035, -13.9574) construction
  line L876 (37.5035, -13.9574) -> (37.5215, -13.9394) construction
  spline S261 degree 3 poles (31.5337, -14.3534) (31.4677, -14.3474) (31.4196, -14.4914) (31.3956, -14.5273) knots 0 0 0 0 1 1 1 1
  line L877 (31.5337, -14.3534) -> (31.4677, -14.3474) construction
  line L878 (31.4677, -14.3474) -> (31.4196, -14.4914) construction
  line L879 (31.4196, -14.4914) -> (31.3956, -14.5273) construction
  spline S262 degree 3 poles (31.3956, -14.5273) (31.2157, -14.8214) (31.0057, -15.0974) (30.7716, -15.3493) knots 1 1 1 1 2 2 2 2
  line L880 (31.3956, -14.5273) -> (31.2157, -14.8214) construction
  line L881 (31.2157, -14.8214) -> (31.0057, -15.0974) construction
  line L882 (31.0057, -15.0974) -> (30.7716, -15.3493) construction
  spline S263 degree 3 poles (30.7716, -15.3493) (30.5317, -15.6133) (30.2316, -15.8953) (29.8657, -15.9793) knots 2 2 2 2 3 3 3 3
  line L883 (30.7716, -15.3493) -> (30.5317, -15.6133) construction
  line L884 (30.5317, -15.6133) -> (30.2316, -15.8953) construction
  line L885 (30.2316, -15.8953) -> (29.8657, -15.9793) construction
  spline S264 degree 3 poles (29.8657, -15.9793) (29.8177, -15.9913) (29.7637, -15.9973) (29.7097, -15.9973) knots 3 3 3 3 4 4 4 4
  line L886 (29.8657, -15.9793) -> (29.8177, -15.9913) construction
  line L887 (29.8177, -15.9913) -> (29.7637, -15.9973) construction
  line L888 (29.7637, -15.9973) -> (29.7097, -15.9973) construction
  spline S265 degree 3 poles (29.7097, -15.9973) (29.6377, -15.9913) (29.5717, -15.9733) (29.5177, -15.9193) knots 4 4 4 4 5 5 5 5
  line L889 (29.7097, -15.9973) -> (29.6377, -15.9913) construction
  line L890 (29.6377, -15.9913) -> (29.5717, -15.9733) construction
  line L891 (29.5717, -15.9733) -> (29.5177, -15.9193) construction
  spline S266 degree 3 poles (29.5177, -15.9193) (29.4877, -15.8893) (29.4577, -15.7873) (29.4217, -15.7693) knots 5 5 5 5 6 6 6 6
  line L892 (29.5177, -15.9193) -> (29.4877, -15.8893) construction
  line L893 (29.4877, -15.8893) -> (29.4577, -15.7873) construction
  line L894 (29.4577, -15.7873) -> (29.4217, -15.7693) construction
  spline S267 degree 3 poles (29.4217, -15.7693) (29.4217, -15.7393) (29.4157, -15.7093) (29.4097, -15.6913) knots 6 6 6 6 7 7 7 7
  line L895 (29.4217, -15.7693) -> (29.4217, -15.7393) construction
  line L896 (29.4217, -15.7393) -> (29.4157, -15.7093) construction
  line L897 (29.4157, -15.7093) -> (29.4097, -15.6913) construction
  line L898 (29.4097, -15.6913) -> (29.3892, -15.6553)
  spline S268 degree 3 poles (29.3892, -15.6553) (29.3831, -15.4753) (29.375, -15.3073) (29.4167, -15.1213) knots 8 8 8 8 9 9 9 9
  line L899 (29.3892, -15.6553) -> (29.3831, -15.4753) construction